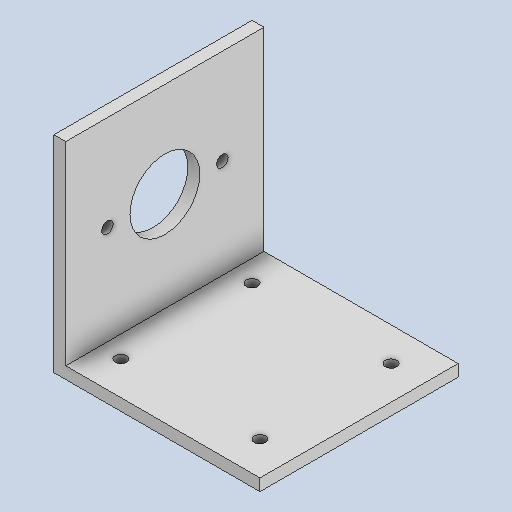
# Autodesk Inventor part: dc motor clamp
Saved by Autodesk Inventor 2022 (Build 260153000, 153)
## iProperties
Created: 2021-07-02
Part Number: dc motor clamp
Material: Generic
Document SubType Name: Sheet Metal
Designer: parag
Density: 1 g/cm^3
Sheet Metal Rule: Default_mm
Appearance: Default
Author: parag
Autodesk Inventor part; units mm, degrees
ref_plane "YZ Plane" through (0, 0, 0) normal (1, 0, 0) x (0, 1, 0)
ref_plane "XZ Plane" through (0, 0, 0) normal (0, 1, 0) x (-1, 0, 0)
ref_plane "XY Plane" through (0, 0, 0) normal (0, 0, 1) x (1, 0, 0)
sketch "Sketch1" plane through (0, 0, 0) normal (0, 0, 1) x (1, 0, 0)
  line L0 (0, 0) -> (0, 52)
  line L1 (0, 52) -> (3, 52)
  line L2 (3, 52) -> (3, 3)
  line L3 (3, 3) -> (52, 3)
  line L4 (52, 3) -> (52, 0)
  line L5 (52, 0) -> (0, 0)
  dimension "d0" = 3
  dimension "d1" = 3
  dimension "d2" = 52
  dimension "d3" = 52
  constraints: 12 end point, 5 perpendicular, 1 vertical
  measures "d0" distance between parallel lines of L2 L0
  measures "d1" distance between parallel lines of L5 L3
  measures "d2" distance between parallel lines of L1 L5
  measures "d3" distance between parallel lines of L4 L0
extrude "Extrusion1" add sketch "Sketch1" along normal blind 50
sketch "Sketch2" plane through (3, 3, 0) normal (1, 0, 0) x (0, 0, -1)
  circle A0 centre (-25, 25) radius 8.8
  line L0 (0, 49) -> (-50, 49) projected
  line L1 (0, 0) -> (0, 49) projected
  circle A1 centre (-10.5, 25) radius 1.4515
  circle A2 centre (-39.5, 25) radius 1.4515
  point P0 (0, -3)
  dimension "d6" = 17.6
  dimension "d7" = 24
  dimension "d8" = 25
  dimension "d9" = 2.903
  dimension "d10" = 2.903
  dimension "d11" = 29
  dimension "d12" = 14.5
  dimension "d13" = 14.5
  constraints: 3 centre point
  measures "d6" diameter of A0
  measures "d7" distance from line of L0 A0.centre
  measures "d8" distance from line of L1 A0.centre
  measures "d9" diameter of A1
  measures "d10" diameter of A2
  measures "d11" distance of A1.centre A2.centre
  measures "d12" distance of A0.centre A1.centre
  measures "d13" distance of A0.centre A2.centre
extrude "Extrusion2" cut sketch "Sketch2" against normal through all
sketch "Sketch3" plane through (3, 3, 0) normal (0, 1, 0) x (1, 0, 0)
  circle A0 centre (5.4515, -41.5485) radius 1.4515
  circle A1 centre (5.4515, -8.4515) radius 1.4515
  circle A2 centre (40.5485, -41.5485) radius 1.4515
  circle A3 centre (40.5485, -8.4515) radius 1.4515
  line L0 (49, -50) -> (0, -50) projected
  line L1 (49, 0) -> (0, 0) projected
  line L2 (49, 0) -> (49, -50) projected
  line L3 (-3, 0) -> (-3, -50) projected
  dimension "d16" = 2.903
  dimension "d17" = 2.903
  dimension "d18" = 2.903
  dimension "d19" = 2.903
  dimension "d20" = 7
  dimension "d21" = 7
  dimension "d22" = 7
  dimension "d23" = 7
  dimension "d24" = 7
  dimension "d25" = 7
  dimension "d26" = 7
  dimension "d27" = 7
  constraints: 4 centre point
  measures "d16" diameter of A0
  measures "d17" diameter of A1
  measures "d18" diameter of A2
  measures "d19" diameter of A3
  measures "d20" distance edge to line of A0 L0
  measures "d21" distance edge to line of A1 L1
  measures "d22" distance edge to line of A2 L0
  measures "d23" distance edge to line of A3 L1
  measures "d24" distance edge to line of A2 L2
  measures "d25" distance edge to line of A3 L2
  measures "d26" distance edge to line of A0 L3
  measures "d27" distance edge to line of A1 L3
extrude "Extrusion3" cut sketch "Sketch3" against normal through all
equation "\"BendRadius\" = Thickness"
equation "\"BendReliefWidth\" = Thickness"
equation "\"BendReliefDepth\" = 0.5 * Thickness"
equation "\"CornerReliefSize\" = 4 * Thickness"
equation "\"MinimumRemnant\" = 2 * Thickness"
equation "\"TransitionRadius\" = BendRadius"
equation "\"JacobiRadiusSize\" = BendRadius"
equation "\"GapSize\" = Thickness"
equation "\"Thickness\" = 0.5"
body "Solid1"
